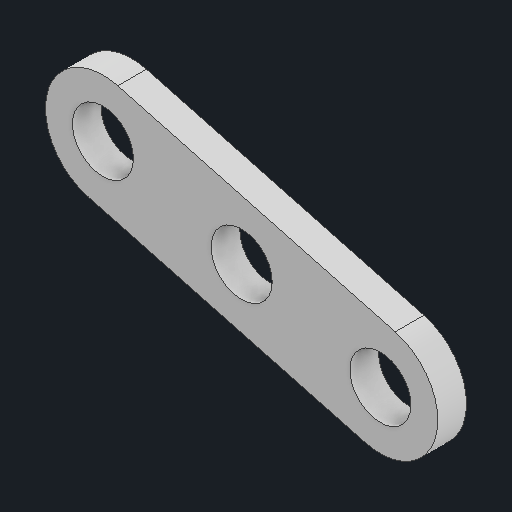
# Autodesk Inventor part: Joiner
Saved by Autodesk Inventor 2023 (Build 270158000, 158)
## iProperties
Created: 2022-06-19
Part Number: Joiner
Material: Generic
Document SubType Name: Modeling
Designer: FizzyApple12
Density: 1 g/cm^3
Appearance: Default
Author: FizzyApple12
Autodesk Inventor part; units mm, degrees
ref_plane "YZ Plane" through (0, 0, 0) normal (1, 0, 0) x (0, 1, 0)
ref_plane "XZ Plane" through (0, 0, 0) normal (0, 1, 0) x (-1, 0, 0)
ref_plane "Work Plane1" through (0, 0, 0) normal (0, 0, 1) x (1, 0, 0)
sketch "Sketch1" plane through (0, 0, 0) normal (0, 0, 1) x (1, 0, 0)
  circle A0 centre (102.5862, 3.8062) radius 3.3782 construction
  line L0 (119.5637, 5.8311) -> (123.8699, 21.902) construction
  line L1 (113.1593, -18.0706) -> (116.2767, -6.4362) construction
  line L2 (116.2767, -6.4362) -> (119.5637, 5.8311) construction
  line L3 (117.9202, -0.3025) -> (102.5862, 3.8062) construction
  line L4 (117.9202, -0.3025) -> (133.2543, -4.4113) construction
  line L5 (133.2543, -4.4113) -> (102.5862, 3.8062) construction
  line L6 (134.8978, 1.7223) -> (104.2297, 9.9398)
  line L7 (100.9427, -2.3274) -> (131.6108, -10.5449)
  arc A1 (131.6108, -10.5449) -> (134.8978, 1.7223) centre (133.2543, -4.4113) ccw
  arc A2 (104.2297, 9.9398) -> (100.9427, -2.3274) centre (102.5862, 3.8062) ccw
  point P0 (0, 0)
  point P1 (117.9202, -0.3025)
  dimension "d0" = 15.875
  dimension "d1" = 12.7
  constraints: 14 end point, 4 point on circle, 4 tangent, 3 coincident, 2 centre point, 2 midpoint, 2 perpendicular, 1 collinear, 1 parallel
  measures "d0" distance of L3.start L4.end
  measures "d1" diameter of A2
extrude "Extrusion1" add sketch "Sketch1" along normal blind 3.175
sketch "Sketch2" plane through (0, 0, 3.175) normal (0, 0, 1) x (1, 0, 0)
  arc A0 (104.2297, 9.9398) -> (100.9427, -2.3274) centre (102.5862, 3.8062) ccw construction
  arc A1 (131.6108, -10.5449) -> (134.8978, 1.7223) centre (133.2543, -4.4113) ccw construction
  line L0 (102.5862, 3.8062) -> (133.2543, -4.4113) construction
  point P0 (0, 0)
  point P1 (117.9202, -0.3025)
  constraints: 2 coincident, 2 end point, 1 midpoint
hole "Hole1" at (102.5862, 3.8062, 3.175) at (117.9202, -0.3025, 3.175) at (133.2543, -4.4113, 3.175) direction (0, 0, -1) diameter 6.7564 depth 13.6144 clearance for "Flat Head Machine Screw (82)" size "1/4" standard "Ansi Unified Screw Threads"
body "Solid1"
